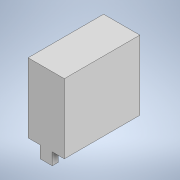
# Autodesk Inventor part: Reload_Motor
Saved by Autodesk Inventor 2020 (Build 240168000, 168)
## iProperties
Created: 2022-03-20
Part Number: Reload_Motor
Material: Generic
Document SubType Name: Modeling
Designer: danie
Density: 1 g/cm^3
Appearance: Default
Author: danie
Autodesk Inventor part; units mm, degrees
ref_plane "YZ Plane" through (0, 0, 0) normal (1, 0, 0) x (0, 1, 0)
ref_plane "XZ Plane" through (0, 0, 0) normal (0, 1, 0) x (-1, 0, 0)
ref_plane "XY Plane" through (0, 0, 0) normal (0, 0, 1) x (1, 0, 0)
sketch "Sketch1" plane through (0, 0, 0) normal (1, 0, 0) x (0, 1, 0)
  line L0 (0, 0) -> (-36.5125, 0)
  line L1 (-36.5125, 0) -> (-36.5125, -39.6875)
  line L2 (-36.5125, -39.6875) -> (0, -39.6875)
  line L3 (0, -39.6875) -> (0, 0)
  dimension "d0" = 36.5125
  dimension "d1" = 39.6875
  constraints: 8 end point, 2 parallel, 1 horizontal, 1 perpendicular
  measures "d0" distance of L2.end L1.end
  measures "d1" distance of L1.end L0.end
extrude "Extrusion1" add sketch "Sketch1" against normal blind 19.05
sketch "Sketch2" plane through (0, -36.5125, -39.6875) normal (0, 0, -1) x (-1, 0, 0)
  line L0 (0, 0) -> (0, 36.5125) construction
  line L1 (0, 0) -> (9.525, 0) construction
  line L2 (0, 0) -> (19.05, 0) construction
  line L3 (0, 0) -> (9.525, 0) construction
  line L4 (9.525, 0) -> (9.525, 1.5875) construction
  line L5 (9.525, 1.5875) -> (9.525, 8.7312) construction
  circle A0 centre (9.525, 8.7312) radius 7.1437
  dimension "d4" = 9.525
  dimension "d5" = 0
  dimension "d6" = 1.5875
  dimension "d7" = 7.1437
  constraints: 8 end point, 2 collinear, 1 coincident, 1 horizontal, 1 perpendicular, 1 vertical, 1 vertical alignment, 2 other
  measures "d4" distance of L0.start L1.end
  measures "d5" distance between parallel lines of L1 L3
  measures "d6" distance of L3.end L4.end
  measures "d7" distance of L4.end L5.end
extrude "Extrusion2" add sketch "Sketch2" along normal blind 2.3813
sketch "Sketch3" plane through (-9.525, -27.7812, -42.0688) normal (0, 0, -1) x (-1, 0, 0)
  circle A0 centre (0, 0) radius 3.175
  point P0 (-9.525, 27.7812)
  dimension "d10" = 6.35
  constraints: 1 centre point
  measures "d10" diameter of A0
extrude "Extrusion3" add sketch "Sketch3" along normal blind 3.9688
sketch "Sketch4" plane through (0, -36.5125, -39.6875) normal (0, -1, 0) x (1, 0, 0)
  line L0 (0, 39.6875) -> (-6.35, 39.6875) construction
  line L1 (0, 39.6875) -> (-19.05, 39.6875) projected
  line L2 (-19.05, 39.6875) -> (-12.7, 39.6875) construction
  line L3 (-6.35, 39.6875) -> (-12.7, 39.6875) construction
  line L4 (-12.7, 39.6875) -> (-12.7, 36.5125)
  line L5 (-12.7, 36.5125) -> (-6.35, 36.5125)
  line L6 (-6.35, 36.5125) -> (-6.35, 39.6875)
  dimension "d13" = 6.35
  dimension "d14" = 6.35
  dimension "d15" = 3.175
  constraints: 12 end point, 2 parallel, 2 point on line, 1 horizontal, 1 perpendicular
  measures "d13" distance of L0.start L0.end
  measures "d14" distance of L1.end L2.end
  measures "d15" distance of L4.end L3.end
extrude "Extrusion4" add sketch "Sketch4" along normal blind 6.35
body "Solid1"
